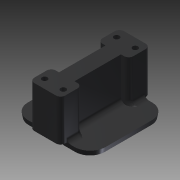
# Autodesk Inventor part: bed_belt
Saved by Autodesk Inventor 2013 (Build 170138000, 138)
## iProperties
Created: 2014-01-31
Part Number: bed_belt
Material: Ogólny
Document SubType Name: Modeling
Designer: Piotr
Density: 1 g/cm^3
Author: Piotr
Autodesk Inventor part; units mm, degrees
ref_plane "YZ Plane" through (0, 0, 0) normal (1, 0, 0) x (0, 1, 0)
ref_plane "XZ Plane" through (0, 0, 0) normal (0, 1, 0) x (-1, 0, 0)
ref_plane "XY Plane" through (0, 0, 0) normal (0, 0, 1) x (1, 0, 0)
sketch "Szkic1" plane through (0, 0, 0) normal (0, 0, 1) x (1, 0, 0)
  line L0 (-25, -25) -> (-10, -25)
  line L1 (25, -25) -> (25, 25)
  line L2 (25, 25) -> (10, 25)
  line L3 (-25, 25) -> (-25, -25)
  line L4 (-25, -25) -> (25, 25) construction
  line L5 (25, -25) -> (-25, 25) construction
  circle A0 centre (-6, 23.25) radius 1.75
  line L6 (0, 25) -> (0, -25) construction
  line L7 (-25, 0) -> (25, 0) construction
  circle A1 centre (6, 23.25) radius 1.75
  circle A2 centre (-6, -23.25) radius 1.75
  circle A3 centre (6, -23.25) radius 1.75
  line L8 (-10, 25) -> (10, 25)
  line L9 (10, 25) -> (10, 15)
  line L10 (10, 15) -> (-10, 15)
  line L11 (-10, 15) -> (-10, 25)
  line L12 (10, -25) -> (10, -15)
  line L13 (10, -15) -> (-10, -15)
  line L14 (-10, -15) -> (-10, -25)
  line L15 (5, -15) -> (-5, -15)
  line L16 (-5, -15) -> (-5, 15)
  line L17 (-5, 15) -> (5, 15)
  line L18 (5, 15) -> (5, -15)
  line L19 (5, -15) -> (-5, 15) construction
  line L20 (-5, -15) -> (5, 15) construction
  line L21 (10, 25) -> (-10, 25)
  line L22 (-10, 25) -> (-25, 25)
  line L23 (-10, -25) -> (10, -25)
  line L24 (10, -25) -> (25, -25)
  line L25 (-10, 25) -> (10, 25)
  line L26 (10, 25) -> (10, 29)
  line L27 (10, 29) -> (-10, 29)
  line L28 (-10, 29) -> (-10, 25)
  line L29 (10, -25) -> (10, -29)
  line L30 (10, -29) -> (-10, -29)
  line L31 (-10, -29) -> (-10, -25)
  line L32 (-10, -25) -> (10, -25)
  point P0 (0, 0)
  point P1 (0, 0)
  dimension "d0" = 50
  dimension "d1" = 50
  dimension "d2" = 3.5
  dimension "d3" = 6
  dimension "d4" = 20
  dimension "d5" = 10
  dimension "d6" = 10
  dimension "d11" = 4
  constraints: 66 end point, 16 parallel, 10 symmetric about line, 8 midpoint, 6 horizontal, 6 perpendicular, 4 centre point, 3 collinear, 3 tangent, 2 point on line, 3 other
  measures "d0" distance of L3.start L1.end
  measures "d1" distance of L1.end L1.start
  measures "d2" diameter of A0
  measures "d3" horizontal distance of point (0, 0) A0.centre
  measures "d4" distance of L2.end L8.start
  measures "d5" distance of L10.end L8.start
  measures "d6" distance of L16.end L17.end
  measures "d11" distance of L25.end L26.end
extrude "Wyciągnięcie proste1" add sketch "Szkic1" against normal blind 3 contours L3 L22 L11 L10 L16 L13 L14 L0 | A2 | A3 | L14 L13 L12 L23 | A1 | A0 | L8 L9 L10 L11 | L16 L10 L18 L13 | L18 L10 L9 L2 L1 L24 L12 L13
extrude "Wyciągnięcie proste2" add sketch "Szkic1" along normal blind 26.8 contours L14 L13 L12 L23 | L23 L29 L30 L31 | L28 L27 L26 L8 | L8 L9 L10 L11 | L16 L10 L18 L13
fillet "Zaokrąglenie1" radius 10 4 edges at (-25, -25, -1.5) (-25, 25, -1.5) (25, -25, -1.5) (25, 25, -1.5)
fillet "Zaokrąglenie2" radius 3 14 edges at (10, 29, 13.4) (10, 15, 13.4) (-10, 29, 13.4) (-10, 15, 13.4) (-10, -15, 13.4) (-10, -29, 13.4) (10, -29, 13.4) (10, -15, 13.4) (-5, 0, 0) (-10, -20, 0) (-10, 20, 0) (10, 20, 0) (5, 0, 0) (10, -20, 0)
chamfer "Faza1" distance 0.5 distance2 3 8 edges at (0, 25, -3) (22.0711, 22.0711, -3) (25, 0, -3) (22.0711, -22.0711, -3) (0, -25, -3) (-22.0711, -22.0711, -3) (-25, 0, -3) (-22.0711, 22.0711, -3) measured on face at (-24.5, 0, -3) measured on face at (0, -24.5, -3) measured on face at (24.5, 0, -3) measured on face at (-21.7175, 21.7175, -3) measured on face at (21.7175, 21.7175, -3) measured on face at (-21.7175, -21.7175, -3) measured on face at (21.7175, -21.7175, -3) measured on face at (0, 24.5, -3)
extrude "Wyciągnięcie proste3" cut sketch "Szkic1" against normal up to next contours A2 | A3 | A1 | A0
